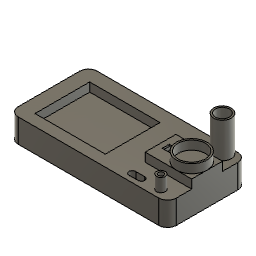
Table Lamp Completed v3 (Autodesk Fusion 360 archive; units mm, degrees)
design "01_Base"
Autodesk Fusion 360 part; units mm, degrees
sketch "Sketch1" plane through (0, 0, 0) normal (0, 1, 0) x (1, 0, 0)
  line L0 (-80, 45) -> (80, 45)
  line L1 (90, 35) -> (90, -35)
  line L2 (80, -45) -> (-80, -45)
  line L3 (-90, -35) -> (-90, 35)
  line L4 (-90, 45) -> (90, -45) construction
  line L5 (90, 45) -> (-90, -45) construction
  arc A0 (-80, 45) -> (-90, 35) centre (-80, 35) ccw
  arc A1 (-90, -35) -> (-80, -45) centre (-80, -35) ccw
  arc A2 (90, 35) -> (80, 45) centre (80, 35) ccw
  arc A3 (80, -45) -> (90, -35) centre (80, -35) ccw
  dimension "d1" = 10
  dimension "d2" = 10
  dimension "d3" = 160
  dimension "d4" = 70
  constraint horizontal L0
  constraint perpendicular L0 L1
  constraint parallel L0 L2
  constraint parallel L1 L3
  constraint coincident L4 origin
  constraint coincident L5 origin
  constraint coincident L4.start L3
  constraint coincident L4.start L0
  constraint tangent L3 A0
  constraint tangent L0 A0
  constraint coincident L5.end L3
  constraint coincident L5.end L2
  constraint tangent L3 A1
  constraint tangent L2 A1
  constraint coincident L5.start L0
  constraint coincident L5.start L1
  constraint tangent L0 A2
  constraint tangent L1 A2
  constraint equal A1 A2
  constraint coincident L4.end L1
  constraint coincident L4.end L2
  constraint tangent L1 A3
  constraint tangent L2 A3
  constraint equal A1 A3
  measures "d1" radius of A0
  measures "d2" radius of A1
  measures "d3" distance of L0.start L0.end
  measures "d4" distance of L1.start L1.end
extrude "Extrude1" add sketch "Sketch1" along normal blind 27
sketch "Sketch2" plane through (0, 27, 0) normal (0, 1, 0) x (-1, 0, 0)
  arc A0 (90, 35) -> (80, 45) centre (80, 35) ccw
  line L0 (80, 45) -> (-80, 45)
  arc A1 (-80, 45) -> (-90, 35) centre (-80, 35) ccw
  line L1 (-90, 35) -> (-90, -35)
  arc A2 (-90, -35) -> (-80, -45) centre (-80, -35) ccw
  line L2 (-80, -45) -> (80, -45)
  arc A3 (80, -45) -> (90, -35) centre (80, -35) ccw
  line L3 (90, -35) -> (90, 35)
  line L4 (73.6586, 32.1311) -> (-6.3414, 32.1311)
  line L5 (-6.3414, 32.1311) -> (-6.3414, -30.0889)
  line L6 (-6.3414, -30.0889) -> (73.6586, -30.0889)
  line L7 (73.6586, -30.0889) -> (73.6586, 32.1311)
  line L8 (73.6586, 32.1311) -> (-6.3414, -30.0889) construction
  line L9 (-6.3414, 32.1311) -> (73.6586, -30.0889) construction
  point P0 (33.6586, 1.0211)
  dimension "d7" = 62.22
  dimension "d8" = 80
  constraint horizontal L4
  constraint perpendicular L4 L5
  constraint parallel L4 L6
  constraint parallel L5 L7
  constraint coincident L8 P0
  constraint coincident L9 P0
  measures "d7" distance of L4.end L5.end
  measures "d8" distance of L5.end L6.end
extrude "Extrude2" cut sketch "Sketch2" against normal blind 10 contours L4 L5 L6 L7
sketch "Sketch3" plane through (0, 27, 0) normal (0, 1, 0) x (-1, 0, 0)
  line L0 (-6.3414, 32.1311) -> (73.6586, 32.1311)
  line L1 (73.6586, 32.1311) -> (73.6586, -30.0889)
  line L2 (73.6586, -30.0889) -> (-6.3414, -30.0889)
  line L3 (-6.3414, -30.0889) -> (-6.3414, 32.1311)
  arc A0 (90, 35) -> (80, 45) centre (80, 35) ccw
  line L4 (80, 45) -> (-80, 45)
  arc A1 (-80, 45) -> (-90, 35) centre (-80, 35) ccw
  line L5 (-90, 35) -> (-90, -35)
  arc A2 (-90, -35) -> (-80, -45) centre (-80, -35) ccw
  line L6 (-80, -45) -> (80, -45)
  arc A3 (80, -45) -> (90, -35) centre (80, -35) ccw
  line L7 (90, -35) -> (90, 35)
  line L8 (-72.5, 0) -> (-72.5, -65) construction
  line L9 (-72.5, -65) -> (-72.5, 75) construction
  line L10 (-72.5, 0) -> (-72.5, 35) construction
  circle A4 centre (-72.5, 35) radius 5
  line L11 (-90, 35) -> (-37, 35) construction
  line L12 (-37, 35) -> (-41.0195, 36.0965) construction
  line L13 (-41.0195, 31.9301) -> (-51.0195, 31.9301)
  line L14 (-41.3547, 39.4001) -> (-51.3367, 39.4001)
  arc A5 (-51.3367, 39.4001) -> (-51.0195, 31.9301) centre (-51.0195, 35.6718) ccw
  circle A6 centre (-72.5, 35) radius 3
  line L15 (-37, 35) -> (-37, 0) construction
  line L16 (-37, 0) -> (-37, -17.5) construction
  line L17 (-90, 0) -> (-90, 17.5) construction
  line L18 (-37, -17.5) -> (-90, -17.5)
  line L19 (-90, -17.5) -> (-90, 17.5)
  line L20 (-90, 17.5) -> (-37, 17.5)
  line L21 (-37, 17.5) -> (-37, -17.5)
  line L22 (-72.5, 0.0486) -> (-72.5, -34.9514)
  circle A7 centre (-72.5, -34.9514) radius 10.0486
  circle A8 centre (-72.5, -34.9514) radius 8.0486
  arc A9 (-41.0195, 31.9301) -> (-41.3547, 39.4001) centre (-40.7065, 35.6867) ccw
  dimension "d13" = 35
  dimension "d14" = 10
  dimension "d15" = 53
  dimension "d22" = -2
  dimension "d26" = 17.5
  dimension "d27" = 17.5
  dimension "d28" = 17.5
  dimension "d47" = 35
  dimension "d48" = -2
  constraint perpendicular L6 L8
  constraint perpendicular L4 L9
  constraint coincident L9 L10.end
  constraint coincident L10.end A4.centre
  constraint coincident A1.end L5.start
  constraint perpendicular L9 L11
  constraint coincident L11.end L12.start
  constraint horizontal L13
  constraint tangent L13 A5
  constraint midpoint L5 L17.start
  constraint horizontal L18
  constraint vertical L19
  constraint horizontal L20
  constraint vertical L21
  constraint coincident L9 L22.start
  constraint perpendicular L18 L22
  constraint coincident L22.end A7.centre
  constraint tangent L6 A7
  constraint parallel L13 L14
  constraint coincident L11.end A9
  measures "d13" distance of L8.start L10.end
  measures "d14" diameter of A4
  measures "d15" distance of A1.end L11.end
  measures "d26" distance of L5 L10.end
  measures "d27" distance of L15.end L16.end
  measures "d28" distance of L17.start L17.end
  measures "d47" distance of L22.start L22.end
extrude "Extrude10" add sketch "Sketch3" along normal blind 40 contours A7
extrude "Extrude8" cut sketch "Sketch3" against normal blind 25 contours L13 L14 A5 A9
extrude "Extrude4" add sketch "Sketch3" along normal blind 10 contours L5 L18 L19 L20 L21
shell "Shell1" thickness 2 removed faces 1 at (26.6667, 0, -15)
extrude "Extrude3" add sketch "Sketch1" along normal blind 2
sketch "Sketch4" plane through (0, 37, 0) normal (0, 1, 0) x (-1, 0, 0)
  line L0 (-37, 17.5) -> (-90, 17.5)
  line L1 (-90, 17.5) -> (-90, -17.5)
  line L2 (-90, -17.5) -> (-37, -17.5)
  line L3 (-37, -17.5) -> (-37, 17.5)
  line L4 (0, 0) -> (-117.4932, 0) construction
  line L5 (-90, 0) -> (-72.5, 0) construction
  circle A0 centre (-72.5, 0) radius 17.5
  circle A1 centre (-72.5, 0) radius 15.5
  line L6 (-43.0004, 0) -> (-43.0004, -4) construction
  line L7 (-43.0004, 0) -> (-43.0004, 4)
  line L8 (-43.0004, 4) -> (-53.0004, 4) construction
  line L9 (-43.0004, -4) -> (-53.0004, -4)
  line L10 (-53.0004, -4) -> (-53.0004, 4)
  line L11 (-53.0004, 4) -> (-43.0004, 4)
  line L12 (-43.0004, 4) -> (-43.0004, -4)
  dimension "d31" = 17.5
  dimension "d32" = -2
  dimension "d33" = 4
  dimension "d34" = 4
  dimension "d35" = 10
  constraint coincident L4.start origin
  constraint perpendicular L1 L4
  constraint midpoint L1 L5.start
  constraint perpendicular L1 L5
  constraint coincident L5.end A0.centre
  constraint coincident L5.start A0
  constraint coincident L4 L6.start
  constraint perpendicular L4 L6
  constraint perpendicular L4 L7
  constraint perpendicular L7 L8
  constraint horizontal L9
  constraint vertical L10
  constraint horizontal L11
  constraint vertical L12
  measures "d31" distance of L5.start L5.end
  measures "d33" distance of L6.start L6.end
  measures "d34" distance of L6.start L7.end
  measures "d35" distance of L7.end L8.end
extrude "Extrude7" add sketch "Sketch4" along normal blind 10 contours A0
extrude "Extrude5" cut sketch "Sketch4" against normal blind 15 contours L7 L9 L10 L11 L12
ref_plane "WorkPlane1" through (63.5, 27, 0) normal (0, 1, 0) x (0, 0, 1)
sketch "Sketch5" plane through (63.5, 27, 0) normal (0, 1, 0) x (1, 0, 0)
  line L0 (-10.4996, 4) -> (-10.4996, -4)
  line L1 (-10.4996, -4) -> (-20.4996, -4)
  line L2 (-20.4996, -4) -> (-20.4996, 4)
  line L3 (-20.4996, 4) -> (-10.4996, 4)
  line L4 (-26.5, -17.5) -> (9, -17.5)
  line L5 (9, 17.5) -> (-26.5, 17.5)
  line L6 (-26.5, 17.5) -> (-26.5, -17.5)
  arc A0 (9, 17.5) -> (9, -17.5) centre (9, 0) ccw
extrude "Extrude11" add sketch "Sketch3" against normal blind 2 contours L5 L18 L19 L20 L21
extrude "Extrude6" add sketch "Sketch5" against normal blind 2 contours L0 L1 L2 L3 | L4 L5 L6 A0
extrude "Extrude9" add sketch "Sketch3" along normal blind 15 contours A4
move_body "Move1" bodies 1 to x (1, 0, 0) y (0, 1, 0) z (0, 0, 1) at (-12.6931, 7.5888, -3.73)

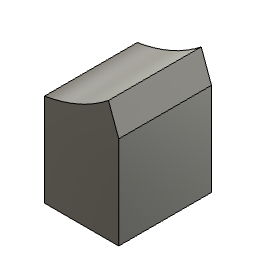
design "Switch"
Autodesk Fusion 360 part; units mm, degrees
sketch "Sketch1" plane through (0, 0, 0) normal (0, 0, 1) x (1, 0, 0)
  line L0 (4, 0) -> (-4, 0) construction
  line L1 (-4, 0) -> (-4, 10) construction
  line L2 (-4, 10) -> (4, 10) construction
  line L3 (4, 10) -> (4, 0)
  line L4 (4, 0) -> (-4, 0)
  line L5 (-4, 0) -> (-4, 10)
  line L6 (4, 10) -> (2.8949, 13.0351)
  arc A0 (-4, 10) -> (2.8949, 13.0351) centre (-6.4022, 24.8064) ccw
  dimension "d1" = 8
  dimension "d2" = 10
  dimension "d4" = 3.23
  dimension "d6" = 15
  constraint horizontal L0
  constraint midpoint origin L0
  constraint perpendicular L0 L1
  constraint horizontal L2
  constraint vertical L3
  constraint horizontal L4
  constraint vertical L5
  measures "d1" distance of L0.start L0.end
  measures "d2" distance of L0.end L1.end
  measures "d4" distance of L2.end L6.end
  measures "d6" radius of A0
extrude "Extrude1" add sketch "Sketch1" along normal blind 10

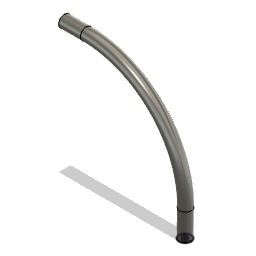
design "Pipe Drawing"
Autodesk Fusion 360 part; units mm, degrees
sketch "Sketch1" plane through (0, 0, 0) normal (0, 0, 1) x (1, 0, 0)
  line L0 (0, 0) -> (1.1636, 67.8107)
  arc A0 (1.1636, 67.8107) -> (-247.84, 321.1235) centre (-247.84, 72.0833) ccw
  line L1 (-247.84, 321.1235) -> (-302.5435, 321.1235)
  constraint tangent A0 L1
  constraint tangent L0 A0
sketch "Sketch2" plane through (0, 0, 0) normal (0, 1, 0) x (1, 0, 0)
  circle A0 centre (0, 0) radius 13
  circle A1 centre (0, 0) radius 15
  dimension "d9" = 26
  dimension "d10" = 2
  constraint coincident A0.centre A1.centre
  measures "d9" diameter of A0
sweep "Sweep1" add profiles "Sketch2" path "Sketch1" along L0 A0 L1 section 1
